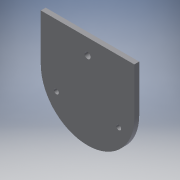
# Autodesk Inventor part: LargeConnectorBodies
Saved by Autodesk Inventor 2016 (Build 200138000, 138)
## iProperties
Created: 2017-03-11
Part Number: LargeConnectorBodies
Material: Generic
Document SubType Name: Modeling
Designer: Owner
Density: 1 g/cm^3
Appearance: Default
Author: Owner
Autodesk Inventor part; units mm, degrees
ref_plane "YZ Plane" through (0, 0, 0) normal (1, 0, 0) x (0, 1, 0)
ref_plane "XZ Plane" through (0, 0, 0) normal (0, 1, 0) x (-1, 0, 0)
ref_plane "XY Plane" through (0, 0, 0) normal (0, 0, 1) x (1, 0, 0)
sketch "Sketch1" plane through (0, 0, 0) normal (0, 0, 1) x (1, 0, 0)
  line L0 (6.35, -214.55) -> (43.1, -214.55) projected
  line L1 (43.1, -214.55) -> (43.1, -189.15) projected
  line L2 (43.1, -189.15) -> (40.1028, -189.15) projected
  line L3 (40.1028, -189.15) -> (40.1028, -176.45) projected
  line L4 (40.1028, -176.45) -> (43.1, -176.45) projected
  line L5 (43.1, -176.45) -> (43.1, -110.25) projected
  line L6 (43.1, -110.25) -> (40.1028, -110.25) projected
  line L7 (40.1028, -110.25) -> (40.1028, -97.55) projected
  line L8 (40.1028, -97.55) -> (43.1, -97.55) projected
  line L9 (43.1, -97.55) -> (43.1, -72.15) projected
  line L10 (43.1, -72.15) -> (35.023, -72.15) projected
  arc A0 (-35.023, -72.15) -> (35.023, -72.15) centre (0, -57.15) ccw projected
  line L11 (-35.023, -72.15) -> (-43.1, -72.15) projected
  line L12 (-43.1, -72.15) -> (-43.1, -97.55) projected
  line L13 (-43.1, -97.55) -> (-40.1028, -97.55) projected
  line L14 (-40.1028, -97.55) -> (-40.1028, -110.25) projected
  line L15 (-40.1028, -110.25) -> (-43.1, -110.25) projected
  line L16 (-43.1, -110.25) -> (-43.1, -176.45) projected
  line L17 (-43.1, -176.45) -> (-40.1028, -176.45) projected
  line L18 (-40.1028, -176.45) -> (-40.1028, -189.15) projected
  line L19 (-40.1028, -189.15) -> (-43.1, -189.15) projected
  line L20 (-43.1, -189.15) -> (-43.1, -214.55) projected
  line L21 (-43.1, -214.55) -> (-6.35, -214.55) projected
  line L22 (-11.16, -143.04) -> (-11.16, -138.135) projected
  line L23 (-11.16, -138.135) -> (10.16, -138.135) projected
  line L24 (10.16, -138.135) -> (10.16, -168.265) projected
  line L25 (10.16, -168.265) -> (-11.16, -168.265) projected
  line L26 (-11.16, -168.265) -> (-11.16, -159.55) projected
  line L27 (-11.16, -159.55) -> (-19.058, -159.55) projected
  line L28 (-19.058, -159.55) -> (-19.058, -164.622) projected
  line L29 (-19.058, -164.622) -> (-22.598, -164.622) projected
  line L30 (-22.598, -164.622) -> (-22.598, -159.55) projected
  line L31 (-22.598, -159.55) -> (-32.258, -159.55) projected
  line L32 (-32.258, -159.55) -> (-32.258, -167.805) projected
  line L33 (-32.258, -167.805) -> (-34.29, -167.805) projected
  line L34 (-34.29, -167.805) -> (-34.29, -159.55) projected
  line L35 (-34.29, -159.55) -> (-38.1, -159.55) projected
  line L36 (-38.1, -159.55) -> (-38.1, -136.69) projected
  line L37 (-38.1, -136.69) -> (-22.598, -136.69) projected
  line L38 (-22.598, -136.69) -> (-22.598, -131.618) projected
  line L39 (-22.598, -131.618) -> (-19.058, -131.618) projected
  line L40 (-19.058, -131.618) -> (-19.058, -136.69) projected
  line L41 (-19.058, -136.69) -> (-15.24, -136.69) projected
  line L42 (-15.24, -136.69) -> (-15.24, -143.04) projected
  arc A1 (-38.1, -57.15) -> (38.1, -57.15) centre (0, -57.15) ccw projected
  line L43 (0, -57.15) -> (0, -82.55)
  circle A2 centre (0, -82.55) radius 38.1
  line L44 (38.1, -82.55) -> (-38.1, -82.55)
  line L45 (-38.1, -82.55) -> (-38.1, -44.45)
  line L46 (-38.1, -44.45) -> (38.1, -44.45)
  line L47 (38.1, -44.45) -> (38.1, -82.55)
  circle A3 centre (25.4, -95.25) radius 1.5 projected
  circle A4 centre (-25.4, -95.25) radius 1.5 projected
  line L48 (-15.24, -143.04) -> (-11.16, -143.04) projected
  line L49 (-6.35, -214.55) -> (-6.35, -203.8154) projected
  line L50 (-6.35, -203.8154) -> (6.35, -203.8154) projected
  line L51 (6.35, -203.8154) -> (6.35, -214.55) projected
  point P0 (0, 0)
  dimension "d1" = 76.2
  dimension "d0" = 25.4
  constraints: 10 end point, 2 parallel, 1 coincident, 1 horizontal, 1 horizontal alignment, 1 perpendicular, 1 vertical, 2 other
  measures "d0" distance of L43.start L43.end
extrude "Extrusion1" add sketch "Sketch1" along normal blind 4 contours L47 A2 L10 | L10 A2 A1 L47 | A2 L44 A0 L10 | L10 A1 A2 | A1 A2 L46 L47 | A2 L44 A0 | A0 L44 A1 A2 | L45 L11 A2 | A2 L11 A0 L44 | A0 L44 | A2 A1 L45 L46 | A2 A1 L11 | L11 L45 A1 A2 | A3 | A4
ref_plane "Work Plane1" through (0, -135.7786, 0) normal (0, 0, 1) x (1, 0, 0)
sketch "Sketch2" plane through (0, 0, 4) normal (0, 0, 1) x (1, 0, 0)
  line L0 (-40.1, -31.75) -> (-43.1, -31.75) projected
  line L1 (-43.1, -31.75) -> (-43.1, -57.15) projected
  line L2 (-43.1, -57.15) -> (-38.1, -57.15) projected
  arc A0 (-38.1, -57.15) -> (38.1, -57.15) centre (0, -57.15) ccw projected
  line L3 (38.1, -57.15) -> (43.1, -57.15) projected
  line L4 (43.1, -57.15) -> (43.1, -31.75) projected
  line L5 (43.1, -31.75) -> (40.1, -31.75) projected
  line L6 (40.1, -31.75) -> (40.1, -19.05) projected
  line L7 (40.1, -19.05) -> (43.1, -19.05) projected
  line L8 (43.1, -19.05) -> (43.1, 24.05) projected
  line L9 (43.1, 24.05) -> (40.1, 24.05) projected
  line L10 (40.1, 24.05) -> (40.1, 36.75) projected
  line L11 (40.1, 36.75) -> (43.1, 36.75) projected
  line L12 (43.1, 36.75) -> (43.1, 62.15) projected
  line L13 (14, 62.15) -> (-14, 62.15) projected
  line L14 (-43.1, 62.15) -> (-43.1, 36.75) projected
  line L15 (-43.1, 36.75) -> (-40.1, 36.75) projected
  line L16 (-40.1, 36.75) -> (-40.1, 24.05) projected
  line L17 (-40.1, 24.05) -> (-43.1, 24.05) projected
  line L18 (-43.1, 24.05) -> (-43.1, -19.05) projected
  line L19 (-43.1, -19.05) -> (-40.1, -19.05) projected
  line L20 (-40.1, -19.05) -> (-40.1, -31.75) projected
  line L21 (15.24, -5.55) -> (11.16, -5.55) projected
  line L22 (11.16, -5.55) -> (11.16, -14.265) projected
  line L23 (11.16, -14.265) -> (-10.16, -14.265) projected
  line L24 (-10.16, -14.265) -> (-10.16, 15.865) projected
  line L25 (-10.16, 15.865) -> (11.16, 15.865) projected
  line L26 (11.16, 15.865) -> (11.16, 7.15) projected
  line L27 (11.16, 7.15) -> (19.058, 7.15) projected
  line L28 (22.598, 7.15) -> (32.266, 7.15) projected
  line L29 (32.266, 7.15) -> (32.266, 15.405) projected
  line L30 (32.266, 15.405) -> (34.282, 15.405) projected
  line L31 (34.282, 15.405) -> (34.282, 7.15) projected
  line L32 (34.282, 7.15) -> (38.1, 7.15) projected
  line L33 (38.1, 7.15) -> (38.1, -15.71) projected
  line L34 (38.1, -15.71) -> (22.598, -15.71) projected
  line L35 (19.058, -15.71) -> (15.24, -15.71) projected
  line L36 (15.24, -15.71) -> (15.24, -5.55) projected
  circle A1 centre (0, -57.15) radius 2.5
  line L37 (19.058, 7.15) -> (19.058, 12.222) projected
  line L38 (19.058, 12.222) -> (22.598, 12.222) projected
  line L39 (22.598, 12.222) -> (22.598, 7.15) projected
  line L40 (22.598, -15.71) -> (22.598, -20.782) projected
  line L41 (22.598, -20.782) -> (19.058, -20.782) projected
  line L42 (19.058, -20.782) -> (19.058, -15.71) projected
  line L43 (-14, 62.15) -> (-14, 31.5) projected
  line L44 (-14, 31.5) -> (-30.4, 31.5) projected
  line L45 (-30.4, 31.5) -> (-30.4, 62.15) projected
  line L46 (-30.4, 62.15) -> (-43.1, 62.15) projected
  line L47 (43.1, 62.15) -> (30.4, 62.15) projected
  line L48 (30.4, 62.15) -> (30.4, 31.5) projected
  line L49 (30.4, 31.5) -> (14, 31.5) projected
  line L50 (14, 31.5) -> (14, 62.15) projected
  point P0 (0, 0)
  dimension "d4" = 5
  constraints: 1 centre point, 1 coincident
  measures "d4" diameter of A1
extrude "Extrusion2" cut sketch "Sketch2" against normal blind 4 contours A1
sketch "Sketch3" plane through (0, 0, 4) normal (0, 0, 1) x (1, 0, 0)
  arc A0 (-35.023, -72.15) -> (35.023, -72.15) centre (0, -57.15) ccw projected
  line L0 (-6.35, -214.55) -> (-6.35, -203.8154) projected
  line L1 (-6.35, -203.8154) -> (6.35, -203.8154) projected
  line L2 (6.35, -203.8154) -> (6.35, -214.55) projected
  line L3 (6.35, -214.55) -> (43.1, -214.55) projected
  line L4 (43.1, -214.55) -> (43.1, -189.15) projected
  line L5 (43.1, -189.15) -> (40.1028, -189.15) projected
  line L6 (40.1028, -189.15) -> (40.1028, -176.45) projected
  line L7 (40.1028, -176.45) -> (43.1, -176.45) projected
  line L8 (43.1, -176.45) -> (43.1, -110.25) projected
  line L9 (43.1, -110.25) -> (40.1028, -110.25) projected
  line L10 (40.1028, -110.25) -> (40.1028, -97.55) projected
  line L11 (40.1028, -97.55) -> (43.1, -97.55) projected
  line L12 (43.1, -97.55) -> (43.1, -72.15) projected
  line L13 (43.1, -72.15) -> (35.023, -72.15) projected
  arc A1 (-35.023, -72.15) -> (35.023, -72.15) centre (0, -57.15) ccw projected
  line L14 (-35.023, -72.15) -> (-43.1, -72.15) projected
  line L15 (-43.1, -72.15) -> (-43.1, -97.55) projected
  line L16 (-43.1, -97.55) -> (-40.1028, -97.55) projected
  line L17 (-40.1028, -97.55) -> (-40.1028, -110.25) projected
  line L18 (-40.1028, -110.25) -> (-43.1, -110.25) projected
  line L19 (-43.1, -110.25) -> (-43.1, -176.45) projected
  line L20 (-43.1, -176.45) -> (-40.1028, -176.45) projected
  line L21 (-40.1028, -176.45) -> (-40.1028, -189.15) projected
  line L22 (-40.1028, -189.15) -> (-43.1, -189.15) projected
  line L23 (-43.1, -189.15) -> (-43.1, -214.55) projected
  line L24 (-43.1, -214.55) -> (-6.35, -214.55) projected
  line L25 (-11.16, -143.04) -> (-11.16, -138.135) projected
  line L26 (-11.16, -138.135) -> (10.16, -138.135) projected
  line L27 (10.16, -138.135) -> (10.16, -168.265) projected
  line L28 (10.16, -168.265) -> (-11.16, -168.265) projected
  line L29 (-11.16, -168.265) -> (-11.16, -159.55) projected
  line L30 (-11.16, -159.55) -> (-19.058, -159.55) projected
  line L31 (-19.058, -159.55) -> (-19.058, -164.622) projected
  line L32 (-19.058, -164.622) -> (-22.598, -164.622) projected
  line L33 (-22.598, -164.622) -> (-22.598, -159.55) projected
  line L34 (-22.598, -159.55) -> (-32.258, -159.55) projected
  line L35 (-32.258, -159.55) -> (-32.258, -167.805) projected
  line L36 (-32.258, -167.805) -> (-34.29, -167.805) projected
  line L37 (-34.29, -167.805) -> (-34.29, -159.55) projected
  line L38 (-34.29, -159.55) -> (-38.1, -159.55) projected
  line L39 (-38.1, -159.55) -> (-38.1, -136.69) projected
  line L40 (-38.1, -136.69) -> (-22.598, -136.69) projected
  line L41 (-22.598, -136.69) -> (-22.598, -131.618) projected
  line L42 (-22.598, -131.618) -> (-19.058, -131.618) projected
  line L43 (-19.058, -131.618) -> (-19.058, -136.69) projected
  line L44 (-19.058, -136.69) -> (-15.24, -136.69) projected
  line L45 (-15.24, -136.69) -> (-15.24, -143.04) projected
  circle A2 centre (0, -57.15) radius 2.5 projected
  arc A3 (-38.1, -82.55) -> (38.1, -82.55) centre (0, -82.55) ccw projected
  line L46 (38.1, -82.55) -> (38.1, -44.45) projected
  line L47 (38.1, -44.45) -> (-38.1, -44.45) projected
  line L48 (-38.1, -44.45) -> (-38.1, -82.55) projected
  line L49 (0, -95.25) -> (25.4, -95.25)
  line L50 (25.4, -95.25) -> (-25.4, -95.25)
  circle A4 centre (25.4, -95.25) radius 2
  circle A5 centre (-25.4, -95.25) radius 2
  circle A6 centre (25.4, -95.25) radius 1.5 projected
  circle A7 centre (-25.4, -95.25) radius 1.5 projected
  line L51 (-15.24, -143.04) -> (-11.16, -143.04) projected
  point P0 (0, 0)
  dimension "d7" = 25.4
  dimension "d8" = 50.8
  dimension "d9" = 4
  dimension "d10" = 4
  constraints: 4 end point, 2 centre point, 2 coincident, 1 horizontal, 1 point on circle, 1 point on line
  measures "d7" distance of L49.start L49.end
  measures "d8" distance of L49.end L50.end
  measures "d9" diameter of A4
  measures "d10" diameter of A5
extrude "Extrusion3" cut sketch "Sketch3" against normal blind 25.4 contours A4 | A5 | A6 | A7
body "Solid1"
